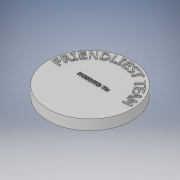
# Autodesk Inventor part: FRIENDLIEST TEAM
Saved by Autodesk Inventor 2018.2 (Build 222227000, 227)
## iProperties
Created: 2018-03-08
Part Number: FRIENDLIEST TEAM
Material: Generic
Document SubType Name: Modeling
Designer: battin.michael
Density: 1 g/cm^3
Appearance: Default
Author: battin.michael
Autodesk Inventor part; units mm, degrees
ref_plane "YZ Plane" through (0, 0, 0) normal (1, 0, 0) x (0, 1, 0)
ref_plane "XZ Plane" through (0, 0, 0) normal (0, 1, 0) x (-1, 0, 0)
ref_plane "XY Plane" through (0, 0, 0) normal (0, 0, 1) x (1, 0, 0)
sketch "Sketch1" plane through (0, 0, 0) normal (0, 1, 0) x (-1, 0, 0)
  circle A0 centre (0, 0) radius 104.775
  dimension "d0" = 209.55
  constraints: 1 centre point, 1 coincident
  measures "d0" diameter of A0
extrude "Extrusion1" add sketch "Sketch1" along normal blind 25.4
sketch "Sketch2" plane through (0, 25.4, 0) normal (0, 1, 0) x (1, 0, 0)
  circle A0 centre (0, 0) radius 104.775
  line L0 (-95.0175, 15.4799) -> (-95.8624, 6.0658)
  line L1 (-95.8624, 6.0658) -> (-90.1549, 5.5535)
  line L2 (-90.1549, 5.5535) -> (-89.3453, 14.574)
  line L3 (-89.3453, 14.574) -> (-86.9508, 14.3591)
  line L4 (-86.9508, 14.3591) -> (-87.7604, 5.3386)
  line L5 (-87.7604, 5.3386) -> (-78.0183, 4.4643)
  line L6 (-78.0183, 4.4643) -> (-78.2597, 1.7745)
  line L7 (-78.2597, 1.7745) -> (-98.4983, 3.5909)
  line L8 (-98.4983, 3.5909) -> (-97.412, 15.6948)
  line L9 (-97.412, 15.6948) -> (-95.0175, 15.4799)
  line L10 (-72.1413, 31.2905) -> (-73.1546, 27.9326)
  line L11 (-73.1546, 27.9326) -> (-82.7504, 24.1203)
  line L12 (-82.7504, 24.1203) -> (-83.6448, 21.1565)
  line L13 (-83.6448, 21.1565) -> (-75.9043, 18.8207)
  line L14 (-75.9043, 18.8207) -> (-76.6845, 16.2353)
  line L15 (-76.6845, 16.2353) -> (-96.1381, 22.1058)
  line L16 (-96.1381, 22.1058) -> (-94.6252, 27.1189)
  spline S0 degree 2 poles (-94.6252, 27.1189) (-94.121, 28.79) (-93.0781, 30.9349) (-92.1067, 31.7598) knots 0 0 0 1 2 2 2
  spline S1 degree 2 poles (-92.1067, 31.7598) (-91.1354, 32.5847) (-88.7134, 33.1438) (-87.1843, 32.6824) knots 0 0 0 1 2 2 2
  spline S2 degree 2 poles (-87.1843, 32.6824) (-85.0561, 32.0401) (-82.8276, 28.994) (-82.6954, 26.9245) knots 0 0 0 1 2 2 2
  line L17 (-82.6954, 26.9245) -> (-72.1413, 31.2905)
  spline S3 degree 2 poles (-87.7928, 29.9248) (-88.6441, 30.1817) (-90.1334, 29.9775) (-90.7493, 29.4753) knots 0 0 0 1 2 2 2
  spline S4 degree 2 poles (-90.7493, 29.4753) (-91.2784, 29.033) (-92.0203, 27.6573) (-92.3438, 26.5853) knots 0 0 0 1 2 2 2
  line L18 (-92.3438, 26.5853) -> (-93.1193, 24.0156)
  line L19 (-93.1193, 24.0156) -> (-85.8045, 21.8083)
  line L20 (-85.8045, 21.8083) -> (-85.1195, 24.0784)
  spline S5 degree 2 poles (-85.1195, 24.0784) (-84.7817, 25.1976) (-84.6382, 27.098) (-85.0675, 27.8983) knots 0 0 0 1 2 2 2
  spline S6 degree 2 poles (-85.0675, 27.8983) (-85.4322, 28.6276) (-86.7839, 29.6203) (-87.7928, 29.9248) knots 0 0 0 1 2 2 2
  line L21 (-67.8473, 38.8917) -> (-71.4138, 31.8749)
  line L22 (-71.4138, 31.8749) -> (-73.2634, 32.8151)
  line L23 (-73.2634, 32.8151) -> (-72.092, 35.1197)
  line L24 (-72.092, 35.1197) -> (-86.5071, 42.4468)
  line L25 (-86.5071, 42.4468) -> (-87.6785, 40.1421)
  line L26 (-87.6785, 40.1421) -> (-89.5281, 41.0823)
  line L27 (-89.5281, 41.0823) -> (-85.9616, 48.099)
  line L28 (-85.9616, 48.099) -> (-84.112, 47.1589)
  line L29 (-84.112, 47.1589) -> (-85.2834, 44.8542)
  line L30 (-85.2834, 44.8542) -> (-70.8683, 37.5271)
  line L31 (-70.8683, 37.5271) -> (-69.6969, 39.8318)
  line L32 (-69.6969, 39.8318) -> (-67.8473, 38.8917)
  line L33 (-66.229, 41.8033) -> (-82.5651, 53.8878)
  line L34 (-82.5651, 53.8878) -> (-75.0049, 64.1077)
  line L35 (-75.0049, 64.1077) -> (-73.0721, 62.678)
  line L36 (-73.0721, 62.678) -> (-79.0262, 54.6291)
  line L37 (-79.0262, 54.6291) -> (-74.5517, 51.3191)
  line L38 (-74.5517, 51.3191) -> (-68.9991, 58.8252)
  line L39 (-68.9991, 58.8252) -> (-67.0663, 57.3954)
  line L40 (-67.0663, 57.3954) -> (-72.6189, 49.8893)
  line L41 (-72.6189, 49.8893) -> (-66.5558, 45.4041)
  line L42 (-66.5558, 45.4041) -> (-60.6017, 53.453)
  line L43 (-60.6017, 53.453) -> (-58.6689, 52.0232)
  line L44 (-58.6689, 52.0232) -> (-66.229, 41.8033)
  line L45 (-45.7174, 63.743) -> (-48.0052, 61.7565)
  line L46 (-48.0052, 61.7565) -> (-66.281, 69.0917)
  line L47 (-66.281, 69.0917) -> (-54.7942, 55.862)
  line L48 (-54.7942, 55.862) -> (-56.6965, 54.2102)
  line L49 (-56.6965, 54.2102) -> (-70.0187, 69.5537)
  line L50 (-70.0187, 69.5537) -> (-67.1216, 72.0692)
  line L51 (-67.1216, 72.0692) -> (-50.3943, 65.2867)
  line L52 (-50.3943, 65.2867) -> (-60.9419, 77.4347)
  line L53 (-60.9419, 77.4347) -> (-59.0395, 79.0865)
  line L54 (-59.0395, 79.0865) -> (-45.7174, 63.743)
  spline S7 degree 2 poles (-32.7399, 82.401) (-31.4662, 79.9267) (-31.4221, 74.9119) (-32.533, 72.9325) knots 0 0 0 1 2 2 2
  spline S8 degree 2 poles (-32.533, 72.9325) (-33.4646, 71.3602) (-35.9888, 69.3201) (-38.1849, 68.1896) knots 0 0 0 1 2 2 2
  line L55 (-38.1849, 68.1896) -> (-42.343, 66.0492)
  line L56 (-42.343, 66.0492) -> (-51.643, 84.116)
  line L57 (-51.643, 84.116) -> (-47.529, 86.2338)
  spline S9 degree 2 poles (-47.529, 86.2338) (-44.9815, 87.5452) (-41.6907, 88.2761) (-40.3191, 88.1301) knots 0 0 0 1 2 2 2
  spline S10 degree 2 poles (-40.3191, 88.1301) (-37.9815, 87.8704) (-34.0965, 85.0364) (-32.7399, 82.401) knots 0 0 0 1 2 2 2
  spline S11 degree 2 poles (-35.2586, 81.1416) (-36.3287, 83.2206) (-39.2198, 85.4549) (-41.011, 85.5886) knots 0 0 0 1 2 2 2
  spline S12 degree 2 poles (-41.011, 85.5886) (-42.2712, 85.6622) (-44.7165, 85.0516) (-46.3416, 84.2151) knots 0 0 0 1 2 2 2
  line L58 (-46.3416, 84.2151) -> (-48.1718, 83.273)
  line L59 (-48.1718, 83.273) -> (-41.012, 69.3642)
  line L60 (-41.012, 69.3642) -> (-39.1819, 70.3063)
  spline S13 degree 2 poles (-39.1819, 70.3063) (-37.5861, 71.1277) (-35.4341, 72.8837) (-34.8074, 74.0768) knots 0 0 0 1 2 2 2
  spline S14 degree 2 poles (-34.8074, 74.0768) (-33.9854, 75.5741) (-34.1733, 79.0333) (-35.2586, 81.1416) knots 0 0 0 1 2 2 2
  line L61 (-13.8837, 77.1687) -> (-25.2436, 74.0747)
  line L62 (-25.2436, 74.0747) -> (-30.5834, 93.6806)
  line L63 (-30.5834, 93.6806) -> (-27.9778, 94.3903)
  line L64 (-27.9778, 94.3903) -> (-23.2698, 77.1041)
  line L65 (-23.2698, 77.1041) -> (-14.5155, 79.4884)
  line L66 (-14.5155, 79.4884) -> (-13.8837, 77.1687)
  line L67 (-4.7131, 78.0615) -> (-12.5362, 77.1932)
  line L68 (-12.5362, 77.1932) -> (-12.7651, 79.2553)
  line L69 (-12.7651, 79.2553) -> (-10.1956, 79.5405)
  line L70 (-10.1956, 79.5405) -> (-11.9795, 95.6122)
  line L71 (-11.9795, 95.6122) -> (-14.549, 95.327)
  line L72 (-14.549, 95.327) -> (-14.7779, 97.3892)
  line L73 (-14.7779, 97.3892) -> (-6.9548, 98.2575)
  line L74 (-6.9548, 98.2575) -> (-6.7259, 96.1953)
  line L75 (-6.7259, 96.1953) -> (-9.2954, 95.9101)
  line L76 (-9.2954, 95.9101) -> (-7.5115, 79.8385)
  line L77 (-7.5115, 79.8385) -> (-4.942, 80.1237)
  line L78 (-4.942, 80.1237) -> (-4.7131, 78.0615)
  line L79 (-1.391, 78.3062) -> (-0.2516, 98.5942)
  line L80 (-0.2516, 98.5942) -> (12.4408, 97.8814)
  line L81 (12.4408, 97.8814) -> (12.306, 95.481)
  line L82 (12.306, 95.481) -> (2.3099, 96.0424)
  line L83 (2.3099, 96.0424) -> (1.9978, 90.4854)
  line L84 (1.9978, 90.4854) -> (11.3198, 89.9619)
  line L85 (11.3198, 89.9619) -> (11.185, 87.5615)
  line L86 (11.185, 87.5615) -> (1.863, 88.0851)
  line L87 (1.863, 88.0851) -> (1.4401, 80.5551)
  line L88 (1.4401, 80.5551) -> (11.4361, 79.9937)
  line L89 (11.4361, 79.9937) -> (11.3013, 77.5934)
  line L90 (11.3013, 77.5934) -> (-1.391, 78.3062)
  spline S15 degree 2 poles (19.5855, 75.2352) (17.4506, 75.7927) (14.6882, 77.4671) (13.5322, 78.4497) knots 0 0 0 1 2 2 2
  line L91 (13.5322, 78.4497) -> (14.3892, 81.7318)
  line L92 (14.3892, 81.7318) -> (14.5804, 81.6819)
  spline S16 degree 2 poles (14.5804, 81.6819) (15.5548, 80.134) (18.4715, 77.9428) (19.9851, 77.5476) knots 0 0 0 1 2 2 2
  spline S17 degree 2 poles (19.9851, 77.5476) (22.1519, 76.9818) (24.8367, 78.2039) (25.2236, 79.6856) knots 0 0 0 1 2 2 2
  spline S18 degree 2 poles (25.2236, 79.6856) (25.5314, 80.8646) (24.7511, 82.6341) (23.5881, 83.3293) knots 0 0 0 1 2 2 2
  spline S19 degree 2 poles (23.5881, 83.3293) (22.7465, 83.8213) (21.3244, 84.567) (20.2681, 85.1492) knots 0 0 0 1 2 2 2
  spline S20 degree 2 poles (20.2681, 85.1492) (19.3192, 85.6863) (17.9221, 86.9191) (17.4713, 87.7346) knots 0 0 0 1 2 2 2
  spline S21 degree 2 poles (17.4713, 87.7346) (17.0365, 88.5459) (16.8249, 90.4732) (17.1245, 91.6203) knots 0 0 0 1 2 2 2
  spline S22 degree 2 poles (17.1245, 91.6203) (17.7485, 94.0102) (22.3213, 96.271) (25.2051, 95.518) knots 0 0 0 1 2 2 2
  spline S23 degree 2 poles (25.2051, 95.518) (26.862, 95.0854) (29.6231, 93.6666) (30.7195, 92.7166) knots 0 0 0 1 2 2 2
  line L93 (30.7195, 92.7166) -> (29.9041, 89.5938)
  line L94 (29.9041, 89.5938) -> (29.7129, 89.6438)
  spline S24 degree 2 poles (29.7129, 89.6438) (28.9975, 90.7496) (26.3987, 92.7897) (24.7896, 93.2098) knots 0 0 0 1 2 2 2
  spline S25 degree 2 poles (24.7896, 93.2098) (22.9732, 93.6841) (20.2816, 92.5659) (19.9197, 91.1798) knots 0 0 0 1 2 2 2
  spline S26 degree 2 poles (19.9197, 91.1798) (19.5952, 89.937) (20.5307, 88.11) (21.686, 87.4509) knots 0 0 0 1 2 2 2
  spline S27 degree 2 poles (21.686, 87.4509) (22.4563, 87.0115) (24.7123, 85.8098) (25.4466, 85.3628) knots 0 0 0 1 2 2 2
  spline S28 degree 2 poles (25.4466, 85.3628) (27.3078, 84.2131) (28.5346, 81.2207) (28.0562, 79.3885) knots 0 0 0 1 2 2 2
  spline S29 degree 2 poles (28.0562, 79.3885) (27.7525, 78.2254) (26.2301, 76.2403) (25.1818, 75.6801) knots 0 0 0 1 2 2 2
  spline S30 degree 2 poles (25.1818, 75.6801) (24.0171, 75.0652) (21.3859, 74.7651) (19.5855, 75.2352) knots 0 0 0 1 2 2 2
  line L95 (33.3718, 70.6299) -> (41.3078, 86.6922)
  line L96 (41.3078, 86.6922) -> (35.1958, 89.712)
  line L97 (35.1958, 89.712) -> (36.2607, 91.8674)
  line L98 (36.2607, 91.8674) -> (50.9058, 84.6317)
  line L99 (50.9058, 84.6317) -> (49.8409, 82.4762)
  line L100 (49.8409, 82.4762) -> (43.7289, 85.496)
  line L101 (43.7289, 85.496) -> (35.793, 69.4337)
  line L102 (35.793, 69.4337) -> (33.3718, 70.6299)
  line L103 (53.896, 56.5463) -> (66.4818, 69.2968)
  line L104 (66.4818, 69.2968) -> (61.6301, 74.0859)
  line L105 (61.6301, 74.0859) -> (63.319, 75.7969)
  line L106 (63.319, 75.7969) -> (74.9444, 64.3215)
  line L107 (74.9444, 64.3215) -> (73.2555, 62.6105)
  line L108 (73.2555, 62.6105) -> (68.4038, 67.3996)
  line L109 (68.4038, 67.3996) -> (55.8179, 54.6492)
  line L110 (55.8179, 54.6492) -> (53.896, 56.5463)
  line L111 (61.7966, 48.1142) -> (78.7075, 59.3803)
  line L112 (78.7075, 59.3803) -> (85.7556, 48.8007)
  line L113 (85.7556, 48.8007) -> (83.7548, 47.4678)
  line L114 (83.7548, 47.4678) -> (78.204, 55.7999)
  line L115 (78.204, 55.7999) -> (73.572, 52.714)
  line L116 (73.572, 52.714) -> (78.7485, 44.9438)
  line L117 (78.7485, 44.9438) -> (76.7477, 43.6108)
  line L118 (76.7477, 43.6108) -> (71.5712, 51.3811)
  line L119 (71.5712, 51.3811) -> (65.2947, 47.1997)
  line L120 (65.2947, 47.1997) -> (70.8456, 38.8676)
  line L121 (70.8456, 38.8676) -> (68.8448, 37.5346)
  line L122 (68.8448, 37.5346) -> (61.7966, 48.1142)
  line L123 (69.3603, 36.9362) -> (90.7726, 38.0924)
  line L124 (90.7726, 38.0924) -> (92.0036, 35.0022)
  line L125 (92.0036, 35.0022) -> (75.6614, 21.1184)
  line L126 (75.6614, 21.1184) -> (74.6072, 23.7649)
  line L127 (74.6072, 23.7649) -> (79.2023, 27.5807)
  line L128 (79.2023, 27.5807) -> (76.3321, 34.7859)
  line L129 (76.3321, 34.7859) -> (70.3719, 34.3968)
  line L130 (70.3719, 34.3968) -> (69.3603, 36.9362)
  line L131 (81.0698, 29.1222) -> (88.7938, 35.5847)
  line L132 (88.7938, 35.5847) -> (78.748, 34.9506)
  line L133 (78.748, 34.9506) -> (81.0698, 29.1222)
  line L134 (78.5695, 1.7631) -> (78.21, 4.4396)
  line L135 (78.21, 4.4396) -> (95.5584, 6.7695)
  line L136 (95.5584, 6.7695) -> (83.0531, 10.4399)
  line L137 (83.0531, 10.4399) -> (82.8339, 12.072)
  line L138 (82.8339, 12.072) -> (93.9343, 18.8628)
  line L139 (93.9343, 18.8628) -> (76.5858, 16.5329)
  line L140 (76.5858, 16.5329) -> (76.2505, 19.0299)
  line L141 (76.2505, 19.0299) -> (96.3897, 21.7346)
  line L142 (96.3897, 21.7346) -> (96.8806, 18.0789)
  line L143 (96.8806, 18.0789) -> (86.3437, 11.5465)
  line L144 (86.3437, 11.5465) -> (98.2089, 8.1888)
  line L145 (98.2089, 8.1888) -> (98.7087, 4.4678)
  line L146 (98.7087, 4.4678) -> (78.5695, 1.7631)
  constraints: 1 centre point, 1 coincident, 1 other
extrude "Extrusion2" add sketch "Sketch2" along normal blind 2.54 contours L0 L1 L2 L3 L4 L5 L6 L7 L8 L9 | L10 L11 L12 L13 L14 L15 L16 S0 S1 S2 L17 | L21 L22 L23 L24 L25 L26 L27 L28 L29 L30 L31 L32 | L33 L34 L35 L36 L37 L38 L39 L40 L41 L42 L43 L44 | L45 L46 L47 L48 L49 L50 L51 L52 L53 L54 | S7 S8 L55 L56 L57 S9 S10 | L61 L62 L63 L64 L65 L66 | L67 L68 L69 L70 L71 L72 L73 L74 L75 L76 L77 L78 | L79 L80 L81 L82 L83 L84 L85 L86 L87 L88 L89 L90 | S15 L91 L92 S16 S17 S18 S19 S20 S21 S22 S23 L93 L94 S24 S25 S26 S27 S28 S29 S30 | L95 L96 L97 L98 L99 L100 L101 L102 | L103 L104 L105 L106 L107 L108 L109 L110 | L111 L112 L113 L114 L115 L116 L117 L118 L119 L120 L121 L122 | L123 L124 L125 L126 L127 L128 L129 L130 | L134 L135 L136 L137 L138 L139 L140 L141 L142 L143 L144 L145 L146
sketch "Sketch3" plane through (0, 25.4, 0) normal (0, 1, 0) x (1, 0, 0)
  line L0 (0, 0) -> (0, 5.5372)
  line L1 (0, 5.5372) -> (104.6286, 5.5372)
  circle A0 centre (0, 0) radius 104.775 projected
  line L2 (-104.6286, 5.5372) -> (104.6286, 5.5372)
  spline S0 degree 2 poles (-32.6567, 10.8601) (-32.6567, 10.3661) (-33.0087, 9.4769) (-33.3236, 9.1681) knots 0 0 0 1 2 2 2
  spline S1 degree 2 poles (-33.3236, 9.1681) (-33.7188, 8.7791) (-34.7871, 8.3777) (-35.6022, 8.3777) knots 0 0 0 1 2 2 2
  line L3 (-35.6022, 8.3777) -> (-36.4605, 8.3777)
  line L4 (-36.4605, 8.3777) -> (-36.4605, 5.5372)
  line L5 (-36.4605, 5.5372) -> (-37.4732, 5.5372)
  line L6 (-37.4732, 5.5372) -> (-37.4732, 13.1572)
  line L7 (-37.4732, 13.1572) -> (-35.559, 13.1572)
  spline S2 degree 2 poles (-35.559, 13.1572) (-34.8797, 13.1572) (-33.9288, 12.9349) (-33.5644, 12.6817) knots 0 0 0 1 2 2 2
  spline S3 degree 2 poles (-33.5644, 12.6817) (-33.1384, 12.3915) (-32.6567, 11.4961) (-32.6567, 10.8601) knots 0 0 0 1 2 2 2
  spline S4 degree 2 poles (-33.7126, 10.8292) (-33.7126, 11.2244) (-33.9843, 11.8049) (-34.2622, 11.9901) knots 0 0 0 1 2 2 2
  spline S5 degree 2 poles (-34.2622, 11.9901) (-34.503, 12.1507) (-35.1452, 12.2803) (-35.6207, 12.2803) knots 0 0 0 1 2 2 2
  line L8 (-35.6207, 12.2803) -> (-36.4605, 12.2803)
  line L9 (-36.4605, 12.2803) -> (-36.4605, 9.2422)
  line L10 (-36.4605, 9.2422) -> (-35.7689, 9.2422)
  spline S6 degree 2 poles (-35.7689, 9.2422) (-35.1514, 9.2422) (-34.3919, 9.4398) (-34.1449, 9.6992) knots 0 0 0 1 2 2 2
  spline S7 degree 2 poles (-34.1449, 9.6992) (-33.9164, 9.9277) (-33.7126, 10.4649) (-33.7126, 10.8292) knots 0 0 0 1 2 2 2
  line L11 (-25.7962, 5.5372) -> (-27.1115, 5.5372)
  line L12 (-27.1115, 5.5372) -> (-29.5198, 8.5691)
  line L13 (-29.5198, 8.5691) -> (-30.6807, 8.5691)
  line L14 (-30.6807, 8.5691) -> (-30.6807, 5.5372)
  line L15 (-30.6807, 5.5372) -> (-31.6934, 5.5372)
  line L16 (-31.6934, 5.5372) -> (-31.6934, 13.1572)
  line L17 (-31.6934, 13.1572) -> (-29.7297, 13.1572)
  spline S8 degree 2 poles (-29.7297, 13.1572) (-29.0752, 13.1572) (-28.1921, 13.0152) (-27.7908, 12.7558) knots 0 0 0 1 2 2 2
  spline S9 degree 2 poles (-27.7908, 12.7558) (-27.3894, 12.4965) (-26.9263, 11.6875) (-26.9263, 11.0886) knots 0 0 0 1 2 2 2
  spline S10 degree 2 poles (-26.9263, 11.0886) (-26.9263, 10.2549) (-27.7784, 9.1249) (-28.5071, 8.8532) knots 0 0 0 1 2 2 2
  line L18 (-28.5071, 8.8532) -> (-25.7962, 5.5372)
  spline S11 degree 2 poles (-27.9822, 11.0083) (-27.9822, 11.3417) (-28.2168, 11.8543) (-28.4638, 12.021) knots 0 0 0 1 2 2 2
  spline S12 degree 2 poles (-28.4638, 12.021) (-28.68, 12.163) (-29.2543, 12.2803) (-29.6742, 12.2803) knots 0 0 0 1 2 2 2
  line L19 (-29.6742, 12.2803) -> (-30.6807, 12.2803)
  line L20 (-30.6807, 12.2803) -> (-30.6807, 9.4151)
  line L21 (-30.6807, 9.4151) -> (-29.7915, 9.4151)
  spline S13 degree 2 poles (-29.7915, 9.4151) (-29.3531, 9.4151) (-28.6553, 9.5695) (-28.4144, 9.8103) knots 0 0 0 1 2 2 2
  spline S14 degree 2 poles (-28.4144, 9.8103) (-28.1921, 10.0203) (-27.9822, 10.6131) (-27.9822, 11.0083) knots 0 0 0 1 2 2 2
  line L22 (-25.1911, 5.5372) -> (-25.1911, 13.1572)
  line L23 (-25.1911, 13.1572) -> (-20.4239, 13.1572)
  line L24 (-20.4239, 13.1572) -> (-20.4239, 12.2556)
  line L25 (-20.4239, 12.2556) -> (-24.1784, 12.2556)
  line L26 (-24.1784, 12.2556) -> (-24.1784, 10.1685)
  line L27 (-24.1784, 10.1685) -> (-20.6771, 10.1685)
  line L28 (-20.6771, 10.1685) -> (-20.6771, 9.2669)
  line L29 (-20.6771, 9.2669) -> (-24.1784, 9.2669)
  line L30 (-24.1784, 9.2669) -> (-24.1784, 6.4388)
  line L31 (-24.1784, 6.4388) -> (-20.4239, 6.4388)
  line L32 (-20.4239, 6.4388) -> (-20.4239, 5.5372)
  line L33 (-20.4239, 5.5372) -> (-25.1911, 5.5372)
  spline S15 degree 2 poles (-17.1882, 5.4013) (-18.0157, 5.4013) (-19.1766, 5.7472) (-19.6891, 5.9942) knots 0 0 0 1 2 2 2
  line L34 (-19.6891, 5.9942) -> (-19.6891, 7.2662)
  line L35 (-19.6891, 7.2662) -> (-19.615, 7.2662)
  spline S16 degree 2 poles (-19.615, 7.2662) (-19.1148, 6.7969) (-17.849, 6.2782) (-17.2623, 6.2782) knots 0 0 0 1 2 2 2
  spline S17 degree 2 poles (-17.2623, 6.2782) (-16.4225, 6.2782) (-15.5642, 6.976) (-15.5642, 7.5503) knots 0 0 0 1 2 2 2
  spline S18 degree 2 poles (-15.5642, 7.5503) (-15.5642, 8.0072) (-16.015, 8.5753) (-16.5028, 8.7173) knots 0 0 0 1 2 2 2
  spline S19 degree 2 poles (-16.5028, 8.7173) (-16.8548, 8.8161) (-17.4414, 8.952) (-17.8798, 9.0631) knots 0 0 0 1 2 2 2
  spline S20 degree 2 poles (-17.8798, 9.0631) (-18.275, 9.1681) (-18.8987, 9.4831) (-19.1395, 9.7362) knots 0 0 0 1 2 2 2
  spline S21 degree 2 poles (-19.1395, 9.7362) (-19.3742, 9.9894) (-19.6335, 10.6687) (-19.6335, 11.1133) knots 0 0 0 1 2 2 2
  spline S22 degree 2 poles (-19.6335, 11.1133) (-19.6335, 12.0395) (-18.1886, 13.2931) (-17.0709, 13.2931) knots 0 0 0 1 2 2 2
  spline S23 degree 2 poles (-17.0709, 13.2931) (-16.4287, 13.2931) (-15.2925, 13.0399) (-14.8047, 12.799) knots 0 0 0 1 2 2 2
  line L36 (-14.8047, 12.799) -> (-14.8047, 11.5887)
  line L37 (-14.8047, 11.5887) -> (-14.8788, 11.5887)
  spline S24 degree 2 poles (-14.8788, 11.5887) (-15.2431, 11.9222) (-16.3793, 12.4162) (-17.003, 12.4162) knots 0 0 0 1 2 2 2
  spline S25 degree 2 poles (-17.003, 12.4162) (-17.7069, 12.4162) (-18.5776, 11.7555) (-18.5776, 11.2182) knots 0 0 0 1 2 2 2
  spline S26 degree 2 poles (-18.5776, 11.2182) (-18.5776, 10.7366) (-18.0651, 10.1623) (-17.5834, 10.0326) knots 0 0 0 1 2 2 2
  spline S27 degree 2 poles (-17.5834, 10.0326) (-17.2623, 9.9462) (-16.3299, 9.7239) (-16.0211, 9.6313) knots 0 0 0 1 2 2 2
  spline S28 degree 2 poles (-16.0211, 9.6313) (-15.2369, 9.3904) (-14.5083, 8.4209) (-14.5083, 7.7108) knots 0 0 0 1 2 2 2
  spline S29 degree 2 poles (-14.5083, 7.7108) (-14.5083, 7.26) (-14.8726, 6.3955) (-15.1999, 6.093) knots 0 0 0 1 2 2 2
  spline S30 degree 2 poles (-15.1999, 6.093) (-15.5642, 5.7595) (-16.4904, 5.4013) (-17.1882, 5.4013) knots 0 0 0 1 2 2 2
  line L38 (-13.477, 5.5372) -> (-13.477, 13.1572)
  line L39 (-13.477, 13.1572) -> (-8.7099, 13.1572)
  line L40 (-8.7099, 13.1572) -> (-8.7099, 12.2556)
  line L41 (-8.7099, 12.2556) -> (-12.4643, 12.2556)
  line L42 (-12.4643, 12.2556) -> (-12.4643, 10.1685)
  line L43 (-12.4643, 10.1685) -> (-8.9631, 10.1685)
  line L44 (-8.9631, 10.1685) -> (-8.9631, 9.2669)
  line L45 (-8.9631, 9.2669) -> (-12.4643, 9.2669)
  line L46 (-12.4643, 9.2669) -> (-12.4643, 6.4388)
  line L47 (-12.4643, 6.4388) -> (-8.7099, 6.4388)
  line L48 (-8.7099, 6.4388) -> (-8.7099, 5.5372)
  line L49 (-8.7099, 5.5372) -> (-13.477, 5.5372)
  line L50 (-2.1458, 5.5372) -> (-3.282, 5.5372)
  line L51 (-3.282, 5.5372) -> (-6.6536, 12.1074)
  line L52 (-6.6536, 12.1074) -> (-6.6536, 5.5372)
  line L53 (-6.6536, 5.5372) -> (-7.5984, 5.5372)
  line L54 (-7.5984, 5.5372) -> (-7.5984, 13.1572)
  line L55 (-7.5984, 13.1572) -> (-6.1596, 13.1572)
  line L56 (-6.1596, 13.1572) -> (-3.0906, 7.1242)
  line L57 (-3.0906, 7.1242) -> (-3.0906, 13.1572)
  line L58 (-3.0906, 13.1572) -> (-2.1458, 13.1572)
  line L59 (-2.1458, 13.1572) -> (-2.1458, 5.5372)
  line L60 (1.1763, 5.5372) -> (1.1763, 12.2556)
  line L61 (1.1763, 12.2556) -> (-1.3801, 12.2556)
  line L62 (-1.3801, 12.2556) -> (-1.3801, 13.1572)
  line L63 (-1.3801, 13.1572) -> (4.7455, 13.1572)
  line L64 (4.7455, 13.1572) -> (4.7455, 12.2556)
  line L65 (4.7455, 12.2556) -> (2.1891, 12.2556)
  line L66 (2.1891, 12.2556) -> (2.1891, 5.5372)
  line L67 (2.1891, 5.5372) -> (1.1763, 5.5372)
  line L68 (5.5236, 5.5372) -> (5.5236, 13.1572)
  line L69 (5.5236, 13.1572) -> (10.2907, 13.1572)
  line L70 (10.2907, 13.1572) -> (10.2907, 12.2556)
  line L71 (10.2907, 12.2556) -> (6.5363, 12.2556)
  line L72 (6.5363, 12.2556) -> (6.5363, 10.1685)
  line L73 (6.5363, 10.1685) -> (10.0375, 10.1685)
  line L74 (10.0375, 10.1685) -> (10.0375, 9.2669)
  line L75 (10.0375, 9.2669) -> (6.5363, 9.2669)
  line L76 (6.5363, 9.2669) -> (6.5363, 6.4388)
  line L77 (6.5363, 6.4388) -> (10.2907, 6.4388)
  line L78 (10.2907, 6.4388) -> (10.2907, 5.5372)
  line L79 (10.2907, 5.5372) -> (5.5236, 5.5372)
  spline S31 degree 2 poles (17.4105, 9.341) (17.4105, 8.2974) (16.5645, 6.6178) (15.8544, 6.1485) knots 0 0 0 1 2 2 2
  spline S32 degree 2 poles (15.8544, 6.1485) (15.274, 5.7842) (14.0822, 5.5372) (13.1559, 5.5372) knots 0 0 0 1 2 2 2
  line L80 (13.1559, 5.5372) -> (11.4022, 5.5372)
  line L81 (11.4022, 5.5372) -> (11.4022, 13.1572)
  line L82 (11.4022, 13.1572) -> (13.1374, 13.1572)
  spline S33 degree 2 poles (13.1374, 13.1572) (14.2119, 13.1572) (15.4345, 12.8361) (15.8668, 12.552) knots 0 0 0 1 2 2 2
  spline S34 degree 2 poles (15.8668, 12.552) (16.6016, 12.0642) (17.4105, 10.4525) (17.4105, 9.341) knots 0 0 0 1 2 2 2
  spline S35 degree 2 poles (16.3546, 9.3534) (16.3546, 10.2302) (15.7741, 11.4714) (15.1999, 11.8234) knots 0 0 0 1 2 2 2
  spline S36 degree 2 poles (15.1999, 11.8234) (14.7923, 12.0642) (13.8722, 12.2803) (13.1868, 12.2803) knots 0 0 0 1 2 2 2
  line L83 (13.1868, 12.2803) -> (12.4149, 12.2803)
  line L84 (12.4149, 12.2803) -> (12.4149, 6.4141)
  line L85 (12.4149, 6.4141) -> (13.1868, 6.4141)
  spline S37 degree 2 poles (13.1868, 6.4141) (13.8599, 6.4141) (14.8788, 6.6302) (15.2925, 6.9204) knots 0 0 0 1 2 2 2
  spline S38 degree 2 poles (15.2925, 6.9204) (15.8235, 7.2786) (16.3546, 8.4642) (16.3546, 9.3534) knots 0 0 0 1 2 2 2
  line L86 (23.5609, 5.5372) -> (23.5609, 12.2556)
  line L87 (23.5609, 12.2556) -> (21.0044, 12.2556)
  line L88 (21.0044, 12.2556) -> (21.0044, 13.1572)
  line L89 (21.0044, 13.1572) -> (27.13, 13.1572)
  line L90 (27.13, 13.1572) -> (27.13, 12.2556)
  line L91 (27.13, 12.2556) -> (24.5736, 12.2556)
  line L92 (24.5736, 12.2556) -> (24.5736, 5.5372)
  line L93 (24.5736, 5.5372) -> (23.5609, 5.5372)
  spline S39 degree 2 poles (33.2989, 12.2865) (33.7312, 11.7802) (34.2128, 10.2982) (34.2128, 9.3472) knots 0 0 0 1 2 2 2
  spline S40 degree 2 poles (34.2128, 9.3472) (34.2128, 8.4209) (33.7435, 6.9204) (33.2989, 6.4141) knots 0 0 0 1 2 2 2
  spline S41 degree 2 poles (33.2989, 6.4141) (32.8296, 5.883) (31.5884, 5.3766) (30.8412, 5.3766) knots 0 0 0 1 2 2 2
  spline S42 degree 2 poles (30.8412, 5.3766) (30.0694, 5.3766) (28.8344, 5.9015) (28.3836, 6.4141) knots 0 0 0 1 2 2 2
  spline S43 degree 2 poles (28.3836, 6.4141) (27.9451, 6.9204) (27.4758, 8.4086) (27.4758, 9.3472) knots 0 0 0 1 2 2 2
  spline S44 degree 2 poles (27.4758, 9.3472) (27.4758, 10.3043) (27.9513, 11.7616) (28.3898, 12.2865) knots 0 0 0 1 2 2 2
  spline S45 degree 2 poles (28.3898, 12.2865) (28.8344, 12.7929) (30.0755, 13.3178) (30.8412, 13.3178) knots 0 0 0 1 2 2 2
  spline S46 degree 2 poles (30.8412, 13.3178) (31.6193, 13.3178) (32.8667, 12.7743) (33.2989, 12.2865) knots 0 0 0 1 2 2 2
  spline S47 degree 2 poles (33.1569, 9.3472) (33.1569, 10.1006) (32.8296, 11.2676) (32.5332, 11.6505) knots 0 0 0 1 2 2 2
  spline S48 degree 2 poles (32.5332, 11.6505) (32.2306, 12.0457) (31.3785, 12.4409) (30.8474, 12.4409) knots 0 0 0 1 2 2 2
  spline S49 degree 2 poles (30.8474, 12.4409) (30.2978, 12.4409) (29.4704, 12.058) (29.1555, 11.6505) knots 0 0 0 1 2 2 2
  spline S50 degree 2 poles (29.1555, 11.6505) (28.8529, 11.2615) (28.5318, 10.0882) (28.5318, 9.3472) knots 0 0 0 1 2 2 2
  spline S51 degree 2 poles (28.5318, 9.3472) (28.5318, 7.8467) (29.7915, 6.2535) (30.8474, 6.2535) knots 0 0 0 1 2 2 2
  spline S52 degree 2 poles (30.8474, 6.2535) (31.9033, 6.2535) (33.1569, 7.8467) (33.1569, 9.3472) knots 0 0 0 1 2 2 2
  line L94 (37.0163, 5.5372) -> (35.7936, 5.5372)
  line L95 (35.7936, 5.5372) -> (35.7936, 6.9945)
  line L96 (35.7936, 6.9945) -> (37.0163, 6.9945)
  line L97 (37.0163, 6.9945) -> (37.0163, 5.5372)
  line L98 (37.0163, 9.798) -> (35.7936, 9.798)
  line L99 (35.7936, 9.798) -> (35.7936, 11.2553)
  line L100 (35.7936, 11.2553) -> (37.0163, 11.2553)
  line L101 (37.0163, 11.2553) -> (37.0163, 9.798)
  dimension "d5" = 5.5372
  constraints: 6 end point, 2 horizontal, 2 point on circle, 1 collinear, 1 point on line, 1 vertical
  measures "d5" distance of L0.start L0.end
extrude "Extrusion3" add sketch "Sketch3" along normal blind 2.54 contours L60 L61 L62 L63 L64 L65 L66 L1 | L2 L51 L52 L54 L55 L56 L57 L58 L59 | L68 L69 L70 L71 L72 L73 L74 L75 L76 L77 L78 L1 | L81 L82 S33 S34 S31 S32 L1 | L2 L38 L39 L40 L41 L42 L43 L44 L45 L46 L47 L48 | L86 L87 L88 L89 L90 L91 L92 L1 | S30 S15 L2 | L2 S15 L34 L35 S16 S17 S18 S19 S20 S21 S22 S23 L36 L37 S24 S25 S26 S27 S28 S29 S30 | S42 S43 S44 S45 S46 S39 S40 S41 L1 | L1 S41 S42 | L2 L22 L23 L24 L25 L26 L27 L28 L29 L30 L31 L32 | L95 L96 L97 L1 | L2 L12 L13 L14 L16 L17 S8 S9 S10 L18 | L6 L7 S2 S3 S0 S1 L3 L4 L2 | L98 L99 L100 L101
body "Solid1"
